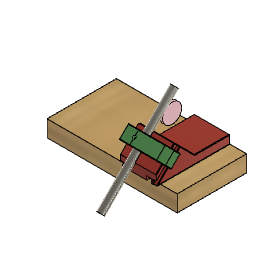
set-screw-keyway-guide (Autodesk Fusion 360 design; units mm, degrees)
Autodesk Fusion 360 part; units mm, degrees
sketch "base" plane through (0, 0, 0) normal (0, 1, 0) x (1, 0, 0) in component "base"
  line L0 (0, 0) -> (50, 0)
  line L1 (45, -5) -> (50, -5)
  line L2 (50, -5) -> (50, 0)
  line L3 (50, 0) -> (45, 0)
  line L4 (45, 0) -> (45, -5)
  line L5 (25.85, -48.5) -> (29.15, -48.5)
  line L6 (29.15, -48.5) -> (29.15, -26.5)
  line L7 (29.15, -26.5) -> (25.85, -26.5)
  line L8 (25.85, -26.5) -> (25.85, -48.5)
  line L9 (29.15, -37.5) -> (-14.7484, -37.5)
  circle A0 centre (27.5, -20.5) radius 4
  circle A1 centre (27.5, -28.5) radius 4
  line L10 (75, 0) -> (-75, 0)
  line L11 (-75, 0) -> (-75, 19)
  line L12 (-75, 19) -> (75, 19)
  line L13 (75, 19) -> (75, 0)
  point P0 (27.5, -26.5)
  point P1 (47.5, -5)
  dimension "d1" = 5
  dimension "d2" = 3.3
  dimension "d3" = 22
  dimension "d4" = 37.5
  dimension "d5" = 45
  dimension "d6" = 20
  dimension "d7" = 8
  dimension "d8" = 6
  dimension "d9" = 8
  dimension "d49" = 19
  dimension "d50" = 150
  dimension "d51" = 25
  constraint coincident L0.start origin
  constraint horizontal L0
  constraint horizontal L1
  constraint vertical L2
  constraint horizontal L3
  constraint vertical L4
  constraint equal L1 L4
  constraint horizontal L5
  constraint vertical L6
  constraint horizontal L7
  constraint vertical L8
  constraint perpendicular L6 L9
  constraint midpoint L6 L9.start
  constraint midpoint L7 P0
  constraint midpoint L1 P1
  constraint vertical P0 A0.centre
  constraint equal A0 A1
  constraint vertical P0 A1.centre
  constraint horizontal L10
  constraint vertical L11
  constraint horizontal L12
  constraint vertical L13
  constraint coincident L0.end L10
  measures "d1" distance of L1.start L1.end
  measures "d2" distance of L5.start L5.end
  measures "d3" distance of L5.start L7.end
  measures "d4" distance of L0 L9
  measures "d5" distance of L0.start L4
  measures "d6" horizontal distance of P0 P1
  measures "d7" diameter of A0
  measures "d8" distance of L7 A0.centre
  measures "d9" distance of A0.centre A1.centre
  measures "d49" distance of L10.end L11.end
  measures "d50" distance of L11.end L12.end
  measures "d51" distance of L0.end L10.start
extrude "Extrude1" add sketch "base" along normal mid plane 80 contours L0 L3 L10 L11 L12 L13 | L0 L1 L2 L3 L4 L10 makes body 1 in component "base"
revolve "Revolve1" add sketch "base" angle 360 about axis through (29.15, 0, 37.5) along (-1, 0, 0) separate body contours L5 L6 L8 L9 makes body 2 in component "base"
sketch "Sketch1" plane through (50, 0, 0) normal (1, 0, 0) x (0, 1, 0) in component "guide"
  line L0 (-40, 0) -> (40, 0) construction
  line L1 (40, 0) -> (40, 5) construction
  line L2 (40, 5) -> (-40, 5) construction
  line L3 (-40, 5) -> (-40, 0) construction
  circle A0 centre (0, 37.5) radius 11 construction
  line L4 (-57.299, -5.6569) -> (6.3406, 57.9828) construction
  line L5 (6.3406, 57.9828) -> (0.6838, 63.6396) construction
  line L6 (0.6838, 63.6396) -> (-62.9558, 0) construction
  line L7 (-62.9558, 0) -> (-57.299, -5.6569) construction
  line L8 (5.6335, 58.6899) -> (-19.0909, 33.9654) construction
  line L9 (3.5122, 60.8112) -> (-60.1274, -2.8284) construction
  line L10 (-45.2548, 0) -> (39.7452, 0)
  line L11 (39.7452, 0) -> (39.7452, 10)
  line L12 (39.7452, 10) -> (-0.7843, 10)
  line L13 (-0.7843, 10) -> (-24.0416, 33.2574)
  line L14 (-45.2548, 12.0442) -> (-24.0416, 33.2574)
  line L15 (-45.2548, 12.0442) -> (-45.2548, 0)
  point P0 (-3.8307, 47.8114)
  point P1 (-10.3114, 41.3307)
  dimension "d164" = 8
  dimension "d165" = 45
  dimension "d166" = 1
  dimension "d167" = 90
  dimension "d171" = 9.1652
  dimension "d172" = 14
  dimension "d175" = 20
  dimension "d176" = 30
  dimension "d178" = 85
  dimension "d179" = 10
  constraint perpendicular L4 L5
  constraint perpendicular L5 L6
  constraint perpendicular L4 L7
  constraint coincident L4.start L7.end
  constraint parallel L4 L8
  constraint tangent A0 L8
  constraint coincident L0 L6.end
  constraint coincident A0 P0
  constraint coincident L4 P0
  constraint coincident A0 P1
  constraint coincident L4 P1
  constraint midpoint L5 L9.start
  constraint midpoint L7 L9.end
  constraint coincident L0 L10.start
  constraint perpendicular L1 L10
  constraint perpendicular L10 L11
  constraint perpendicular L1 L12
  constraint coincident L9 L13.end
  constraint perpendicular L9 L13
  constraint coincident L9 L14.start
  constraint vertical L15
  constraint coincident L10.start L15.end
  measures "d164" distance of L4.end L5.end
  measures "d165" angle of L2 L4
  measures "d166" distance of L4 L8
  measures "d167" distance of L5.end L6.end
  measures "d171" distance of P0 P1
  measures "d172" distance of A0.centre L9
  measures "d175" distance of A0.centre L13
  measures "d176" distance of L13.end L14.start
  measures "d178" distance of L10.start L10.end
  measures "d179" distance of L10.end L11.end
extrude "Extrude1'" add sketch "Sketch1" along normal blind 6 and the other way blind 35 separate body makes body 3 in component "guide"
sketch "Sketch2" plane through (0.1164, 4.3012, 4.9145) normal (0, 0.707107, 0.707107) x (-1, 0, 0) in component "guide"
  line L0 (-25.7336, 15.0828) -> (-25.7336, 37.0828) construction
  line L1 (-29.0336, 15.0828) -> (-29.0336, 37.0828) construction
  line L2 (-14.8836, 40.0828) -> (-55.8836, 40.0828)
  line L3 (-55.8836, 40.0828) -> (-55.8836, 7.1919)
  line L4 (-55.8836, 7.1919) -> (-14.8836, 7.1919) construction
  line L5 (-14.8836, 7.1919) -> (-14.8836, 40.0828)
  line L6 (-25.7336, 37.0828) -> (-29.0336, 37.0828)
  line L7 (-27.3836, 37.0828) -> (-27.3836, 40.0828) construction
  circle A0 centre (-27.3836, 40.0828) radius 4 construction
  arc A1 (-31.6336, 40.0828) -> (-23.1336, 40.0828) centre (-27.3836, 40.0828) ccw
  line L8 (-55.8836, 35.0828) -> (-51.8836, 35.0828)
  line L9 (-51.8836, 35.0828) -> (-51.8836, 31.0828)
  line L10 (-51.8836, 31.0828) -> (-55.8836, 31.0828)
  line L11 (-35.3836, 40.0828) -> (-35.3836, 29.0249) construction
  line L12 (-18.8836, 31.0828) -> (-14.8836, 31.0828)
  line L13 (-18.8836, 35.0828) -> (-18.8836, 31.0828)
  line L14 (-14.8836, 35.0828) -> (-18.8836, 35.0828)
  dimension "d184" = 8
  dimension "d185" = 0.25
  dimension "d186" = 4
  dimension "d187" = 4
  dimension "d188" = 5
  constraint coincident L0.end L6.start
  constraint coincident L1.end L6.end
  constraint midpoint L6 L7.start
  constraint coincident L2 L7.end
  constraint perpendicular L2 L7
  constraint coincident L7.end A0.centre
  constraint coincident L2 A1.end
  constraint coincident L2 A1.start
  constraint coincident L3 L8.start
  constraint perpendicular L3 L8
  constraint perpendicular L8 L9
  constraint perpendicular L3 L10
  constraint coincident L3 L10.end
  constraint midpoint L2 L11.start
  constraint perpendicular L2 L11
  constraint symmetric L8.start L11 L14.start
  constraint symmetric L8.end L11 L13.start
  constraint symmetric L9.end L11 L12.start
  constraint symmetric L10.end L11 L12.end
  measures "d184" diameter of A0
  measures "d185" distance of A0 A1
  measures "d186" distance of L8.end L9.end
  measures "d187" distance of L8.start L8.end
  measures "d188" distance of L2 L8
extrude "Extrude2" cut sketch "Sketch2" against normal through all bodies 3 in component "guide"
sketch "Sketch3" plane through (0, -45.2548, 0) normal (0, -1, 0) x (1, 0, 0) in component "guide"
  line L0 (15, 0.8) -> (19.7088, 0.8)
  line L1 (19.7088, 0.8) -> (20, 0)
  line L2 (25, 0) -> (25.2912, 0.8)
  line L3 (25.2912, 0.8) -> (44.6, 0.8)
  line L4 (44.6, 0.8) -> (44.6, 5.6)
  line L5 (44.6, 5.6) -> (50.4, 5.6)
  line L6 (50.4, 5.6) -> (50.4, 0.8)
  line L7 (50.4, 0.8) -> (50.6912, 0)
  line L8 (45, 5) -> (45, 0) construction
  line L9 (50, 0) -> (50, 5) construction
  line L10 (50, 5) -> (45, 5) construction
  line L11 (19, 4.9731) -> (19, 0) construction
  line L12 (19, 0) -> (52, 0)
  line L13 (52, 0) -> (52, 4.9731) construction
  line L14 (52, 4.9731) -> (56, 4.9731)
  line L15 (56, 4.9731) -> (56, 0)
  line L16 (15, 4.9731) -> (15, 0)
  line L17 (19, 0) -> (15, 0)
  line L18 (52, 0) -> (56, 0)
  line L19 (55.7088, 0) -> (56, 0.8)
  line L20 (15, 4.9731) -> (15, 12.0442)
  dimension "d191" = 5
  dimension "d227" = 0.8
  dimension "d228" = 70
  dimension "d229" = 70
  dimension "d230" = 70
  dimension "d232" = 0.4
  dimension "d233" = 0.4
  dimension "d234" = 0.6
  dimension "d236" = 70
  constraint perpendicular L3 L4
  constraint perpendicular L4 L5
  constraint perpendicular L5 L6
  constraint coincident L3 L6.end
  constraint collinear L0 L3
  constraint horizontal L3
  constraint coincident L1.end L12
  constraint coincident L2.start L12
  constraint coincident L7.end L12
  constraint perpendicular L14 L15
  constraint vertical L16
  constraint coincident L0.start L16
  constraint coincident L11.end L12.start
  constraint coincident L16 L17.end
  constraint perpendicular L16 L17
  constraint coincident L12.end L13.start
  constraint coincident L15 L18.end
  constraint perpendicular L15 L18
  constraint coincident L14.end L15.start
  constraint coincident L15.end L18.end
  constraint coincident L18 L19.start
  constraint coincident L15 L19.end
  constraint coincident L3 L19.end
  constraint coincident L16.start L20.start
  constraint coincident L16.end L17.end
  measures "d191" distance of L1.end L2.start
  measures "d227" distance of L3 L12
  measures "d228" angle of L1 L12
  measures "d229" angle of L2 L12
  measures "d230" angle of L7 L12
  measures "d232" distance of L6 L9
  measures "d233" distance of L4 L8
  measures "d234" distance of L5 L10
  measures "d236" angle of L18 L19
extrude "Extrude4" cut sketch "Sketch3" against normal through all bodies 3 in component "guide"
chamfer "Chamfer1" distance 0.6 angle 45 44 edges at (34.9456, -45.2548, 0.8) (51.3456, -45.2548, 0) (25.1456, -45.2548, 0.4) (22.5, -45.2548, 0) (19.8544, -45.2548, 0.4) (19.3544, -45.2548, 0.8) (53.8544, -44.5711, 0) (52, -45.2548, 2.4865) (54, -45.2548, 4.9731) (19, -45.2548, 2.8865) (17, -45.2548, 4.9731) (43.875, -24.0416, 33.2574) (56, -22.2739, 31.4896) (52, -19.0919, 28.3076) (54, -20.5061, 29.7218) (54, -17.6777, 26.8934) (56, -9.231, 18.4467) (27.5, -21.0364, 30.2522) (19.125, -24.0416, 33.2574) (15, -22.2739, 31.4896) (17, -20.5061, 29.7218) (19, -19.0919, 28.3076) (17, -17.6777, 26.8934) (15, -9.231, 18.4467) (56, 19.4804, 10) (35.5, 39.7452, 10) (15, 19.4804, 10) (56, 39.7452, 5.4) (15, 39.7452, 5.4) (17.3544, 39.7452, 0.8) (19.8544, 39.7452, 0.4) (25.1456, 39.7452, 0.4) (22.5, 39.7452, 0) (34.9456, 39.7452, 0.8) (53.2, 39.7452, 0) (50.5456, 39.7452, 0.4) (50.4, 39.7452, 3.2) (47.5, 39.7452, 5.6) (44.6, 39.7452, 3.2) (56, -30.7244, 13.8467) (56, -34.6482, 22.6508) (56, -32.8805, 17.3475) (15, -30.7244, 13.8467) (15, -32.8805, 17.3475) on bodies 3 in component "guide"
sketch "Sketch1 (2)" plane through (0, 4.6079, 4.6079) normal (0, 0.707107, 0.707107) x (-1, 0, 0) in component "clamp"
  line L0 (-55.4, 7.6256) -> (-15.6, 7.6256) construction
  line L1 (-59.4, 31.9165) -> (-52.4, 31.9165)
  line L2 (-52.4, 31.9165) -> (-52.4, 35.2665)
  line L3 (-52.4, 35.2665) -> (-56.4, 35.2665)
  line L4 (-56.4, 35.2665) -> (-56.4, 43.5165)
  arc A0 (-54.4, 45.5165) -> (-56.4, 43.5165) centre (-54.4, 43.5165) ccw
  arc A1 (-61.4, 33.9165) -> (-59.4, 31.9165) centre (-59.4, 33.9165) ccw
  line L5 (-61.4, 33.9165) -> (-61.4, 43.5165)
  arc A2 (-55.9422, 50.3445) -> (-61.4, 43.5165) centre (-54.4, 43.5165) ccw
  line L6 (-35.5, 7.6256) -> (-35.5, 23.0556) construction
  line L7 (-14.6, 35.2665) -> (-14.6, 43.5165)
  line L8 (-9.6, 33.9165) -> (-9.6, 43.5165)
  arc A3 (-9.6, 43.5165) -> (-13.0181, 49.5307) centre (-16.6, 43.5165) ccw
  arc A4 (-11.6, 31.9165) -> (-9.6, 33.9165) centre (-11.6, 33.9165) ccw
  line L9 (-11.6, 31.9165) -> (-18.6, 31.9165)
  line L10 (-18.6, 31.9165) -> (-18.6, 35.2665)
  line L11 (-18.6, 35.2665) -> (-14.6, 35.2665)
  arc A5 (-14.6, 43.5165) -> (-16.6, 45.5165) centre (-16.6, 43.5165) ccw
  circle A6 centre (-27.5, 40.5165) radius 4 construction
  line L12 (-27.5, 40.5165) -> (-27.5, 53.5165) construction
  line L13 (-54.4, 45.5165) -> (-16.6, 45.5165)
  arc A7 (-13.0181, 49.5307) -> (-27.5, 53.5165) centre (-27.5, 25.2148) ccw
  arc A8 (-27.5, 53.5165) -> (-55.9422, 50.3445) centre (-27.5, -75.5852) ccw
  line L14 (-55.4, 30.9165) -> (-55.4, 7.6256)
  line L15 (-15.6, 7.6256) -> (-15.6, 30.9165)
  line L16 (-15.6, 30.9165) -> (-19.6, 30.9165)
  line L17 (-19.6, 30.9165) -> (-19.6, 36.1165)
  line L18 (-19.6, 36.1165) -> (-15.6, 36.1165)
  line L19 (-15.6, 36.1165) -> (-15.6, 39.9165)
  line L20 (-15.6, 39.9165) -> (-22.6873, 39.9165)
  arc A9 (-32.3127, 39.9165) -> (-22.6873, 39.9165) centre (-27.5, 40.5165) ccw
  line L21 (-32.3127, 39.9165) -> (-55.4, 39.9165)
  line L22 (-55.4, 39.9165) -> (-55.4, 36.1165)
  line L23 (-55.4, 36.1165) -> (-51.4, 36.1165)
  line L24 (-51.4, 36.1165) -> (-51.4, 30.9165)
  line L25 (-51.4, 30.9165) -> (-55.4, 30.9165)
  dimension "d205" = 5
  dimension "d206" = 2
  dimension "d207" = 2
  dimension "d208" = 8
  dimension "d210" = 8
  constraint perpendicular L1 L2
  constraint perpendicular L3 L4
  constraint tangent L4 A0
  constraint tangent L1 A1
  constraint perpendicular L1 L5
  constraint tangent L5 A2
  constraint tangent A1 L5
  constraint coincident A0.centre A2.centre
  constraint midpoint L0 L6.start
  constraint perpendicular L0 L6
  constraint symmetric L1.start L6 A4.start
  constraint symmetric L1.end L6 L9.end
  constraint symmetric L2.end L6 L10.end
  constraint symmetric L3.end L6 L7.start
  constraint symmetric L4.end L6 L7.end
  constraint symmetric A0.start L6 A5.end
  constraint symmetric A0 L6 A5
  constraint symmetric A1.start L6 L8.start
  constraint symmetric A1 L6 A4
  constraint symmetric L5.end L6 L8.end
  constraint symmetric A2 L6 A3
  constraint vertical L12
  constraint tangent A5 L13
  constraint coincident L12 A7.centre
  constraint tangent A3 A7
  constraint coincident L12 A8.centre
  constraint tangent A2 A8
  measures "d205" distance of L4 L5
  measures "d206" radius of A1
  measures "d207" radius of A0
  measures "d208" diameter of A6
  measures "d210" distance of L12.end L13
extrude "Extrude1''" add sketch "Sketch1 (2)" against normal blind 15 from surface at -5 separate body makes body 4 in component "clamp"
sketch "Sketch3 (2)" plane through (0, -32.185, 32.185) normal (0, 0.707107, -0.707107) x (-1, 0, 0) in component "clamp"
  line L0 (-16.6, 1.5165) -> (-54.4, 1.5165)
  line L1 (-54.4, 1.5165) -> (-54.4, -13.4835) construction
  line L2 (-54.4, -13.4835) -> (-16.6, -13.4835) construction
  line L3 (-16.6, -13.4835) -> (-16.6, 1.5165) construction
  line L4 (-23.25, 5.9165) -> (-23.25, -23.4835) construction
  line L5 (-16.6, -5.9835) -> (-27.5, -5.9835) construction
  line L6 (-27.5, -5.9835) -> (-27.5, 4.7862) construction
  circle A0 centre (-27.5, -5.9835) radius 1.9
  line L7 (-30.65, 1.5165) -> (-30.65, -7.2248)
  line L8 (-30.65, -7.2248) -> (-27.5, -9.0435)
  line L9 (-27.5, -9.0435) -> (-24.35, -7.2248)
  line L10 (-24.35, -7.2248) -> (-24.35, 1.5165)
  line L11 (-28.825, -8.2785) -> (-27.5, -5.9835)
  line L12 (-23.25, -23.4835) -> (-23.25, 5.9165)
  line L13 (-31.75, 5.9165) -> (-31.75, -23.4835)
  dimension "d214" = 3.8
  dimension "d215" = 120
  dimension "d216" = 2.65
  dimension "d217" = 6.3
  constraint midpoint L3 L5.start
  constraint perpendicular L5 L6
  constraint coincident L5.end L6.start
  constraint coincident L0 L7.start
  constraint perpendicular L0 L7
  constraint coincident L0 L10.end
  constraint perpendicular L0 L10
  constraint symmetric L6 L7.end L9.end
  constraint coincident L6 L8.end
  constraint coincident L8 L11.start
  constraint perpendicular L8 L11
  constraint symmetric L4.start L6 L13.start
  measures "d214" diameter of A0
  measures "d215" angle of L8 L9
  measures "d216" distance of L11.start L5.end
  measures "d217" distance of L7 L10
extrude "Extrude2'" cut sketch "Sketch3 (2)" against normal through all contours A0 bodies 4 in component "clamp"
extrude "Extrude3" cut sketch "Sketch3 (2)" against normal blind 3.2 from surface at -1 bodies 4 in component "clamp"
chamfer "Chamfer1'" distance 0.6 angle 45 19 edges at (35.5, -31.1127, 33.2574) (55.8142, -30.6985, 32.8431) (56.4, -26.7817, 28.9263) (14.6, -26.7817, 28.9263) (15.1858, -30.6985, 32.8431) (16.6, -23.8649, 26.0095) (18.6, -22.6805, 24.8251) (15.1, -21.496, 23.6407) (10.1858, -21.9103, 24.0549) (9.6, -26.3044, 28.449) (10.5142, -32.1442, 34.2889) (19.9898, -36.0521, 38.1967) (41.8092, -36.2071, 38.3517) (59.8679, -32.789, 34.9337) (61.4, -26.3044, 28.449) (60.8142, -21.9103, 24.0549) (55.9, -21.496, 23.6407) (52.4, -22.6805, 24.8251) (54.4, -23.8649, 26.0095) on bodies 4 in component "clamp"
chamfer "Chamfer1'" distance 0.6 angle 45 1 faces at (39.1828, -43.2719, 24.2033) on bodies 4 in component "clamp"
sketch "Sketch1 (3)" plane through (0, 4.6079, 4.6079) normal (0, 0.707107, 0.707107) x (-1, 0, 0) in component "workpiece"
  circle A0 centre (-27.5, 40.5165) radius 4
  arc A1 (-31.75, 40.5165) -> (-23.25, 40.5165) centre (-27.5, 40.5165) ccw
  dimension "d222" = 8
  constraint coincident A0.centre A1.centre
  measures "d222" diameter of A0
extrude "Extrude1'''" add sketch "Sketch1 (3)" along normal blind 40 and the other way blind 80 separate body makes body 5 in component "workpiece"
component "base" placed x (1, 0, 0) y (0, 1, 0) z (0, 0, 1) at (0, 0, 0)
component "guide" placed x (1, 0, 0) y (0, 1, 0) z (0, 0, 1) at (0, 0, 0)
component "clamp" placed x (1, 0, 0) y (0, 1, 0) z (0, 0, 1) at (0, 0, 0)
component "workpiece" placed x (1, 0, 0) y (0, 1, 0) z (0, 0, 1) at (0, 0, 0)
equation "fit_clearance = 0.25 mm"
equation "run_clearance = 0.4 mm"
equation "d185 = fit_clearance"
equation "d214 = 3 mm + 2 * run_clearance"
equation "d216 = 2.25 mm + run_clearance"
equation "d217 = 5.5 mm + 2 * run_clearance"
equation "d220 = -2.4 mm - 2 * run_clearance"
equation "d229 = d228"
equation "d230 = d228"
equation "d232 = run_clearance"
equation "d233 = run_clearance"
equation "d234 = run_clearance * 1.5"
equation "d236 = d228"
